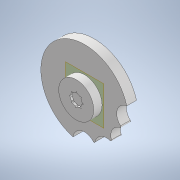
# Autodesk Inventor part: handle_base3
Saved by Autodesk Inventor 2021 (Build 250183000, 183)
## iProperties
Created: 2021-07-05
Part Number: handle_base3
Material: Generic
Document SubType Name: Modeling
Designer: teh18
Density: 1 g/cm^3
Appearance: Default
Author: teh18
Autodesk Inventor part; units mm, degrees
ref_plane "YZ Plane" through (0, 0, 0) normal (1, 0, 0) x (0, 1, 0)
ref_plane "XZ Plane" through (0, 0, 0) normal (0, 1, 0) x (-1, 0, 0)
ref_plane "XY Plane" through (0, 0, 0) normal (0, 0, 1) x (1, 0, 0)
sketch "Sketch1" plane through (0, 0, 0) normal (0, 0, 1) x (1, 0, 0)
  circle A0 centre (0, 0) radius 6
  circle A1 centre (0, 0) radius 20 projected
  circle A2 centre (0, 0) radius 5 projected
  arc A3 (6.0947, -0.2544) -> (5.2397, 3.1233) centre (0, 0) ccw projected
  arc A4 (4.1297, -4.4895) -> (5.9136, -1.4965) centre (0, 0) ccw projected
  arc A5 (-0.2544, -6.0947) -> (3.1233, -5.2397) centre (0, 0) ccw projected
  arc A6 (-4.4895, -4.1297) -> (-1.4965, -5.9136) centre (0, 0) ccw projected
  arc A7 (-6.0947, 0.2544) -> (-5.2397, -3.1233) centre (0, 0) ccw projected
  arc A8 (-4.1297, 4.4895) -> (-5.9136, 1.4965) centre (0, 0) ccw projected
  arc A9 (0.2544, 6.0947) -> (-3.1233, 5.2397) centre (0, 0) ccw projected
  arc A10 (4.4895, 4.1297) -> (1.4965, 5.9136) centre (0, 0) ccw projected
  line L0 (5.7362, 4.2762) -> (5.2397, 3.1233) projected
  line L1 (6.0947, -0.2544) -> (7.0798, -1.0323) projected
  line L2 (7.0798, -1.0323) -> (5.9136, -1.4965) projected
  line L3 (4.1297, -4.4895) -> (4.2762, -5.7362) projected
  line L4 (4.2762, -5.7362) -> (3.1233, -5.2397) projected
  line L5 (-0.2544, -6.0947) -> (-1.0323, -7.0798) projected
  line L6 (-1.0323, -7.0798) -> (-1.4965, -5.9136) projected
  line L7 (-4.4895, -4.1297) -> (-5.7362, -4.2762) projected
  line L8 (-5.7362, -4.2762) -> (-5.2397, -3.1233) projected
  line L9 (-6.0947, 0.2544) -> (-7.0798, 1.0323) projected
  line L10 (-7.0798, 1.0323) -> (-5.9136, 1.4965) projected
  line L11 (-4.1297, 4.4895) -> (-4.2762, 5.7362) projected
  line L12 (-4.2762, 5.7362) -> (-3.1233, 5.2397) projected
  line L13 (0.2544, 6.0947) -> (1.0323, 7.0798) projected
  line L14 (1.0323, 7.0798) -> (1.4965, 5.9136) projected
  line L15 (4.4895, 4.1297) -> (5.7362, 4.2762) projected
  line L16 (4.1567, -5.5758) -> (4.0244, -4.4502)
  arc A11 (4.0244, -4.4502) -> (5.8289, -1.4226) centre (0, 0) ccw
  line L17 (5.8289, -1.4226) -> (6.8819, -1.0035)
  line L18 (6.8819, -1.0035) -> (5.9924, -0.3011)
  arc A12 (5.9924, -0.3011) -> (5.1276, 3.1157) centre (0, 0) ccw
  line L19 (5.1276, 3.1157) -> (5.5758, 4.1567)
  line L20 (5.5758, 4.1567) -> (4.4502, 4.0244)
  arc A13 (4.4502, 4.0244) -> (1.4226, 5.8289) centre (0, 0) ccw
  line L21 (1.4226, 5.8289) -> (1.0035, 6.8819)
  line L22 (1.0035, 6.8819) -> (0.3011, 5.9924)
  arc A14 (0.3011, 5.9924) -> (-3.1157, 5.1276) centre (0, 0) ccw
  line L23 (-3.1157, 5.1276) -> (-4.1567, 5.5758)
  line L24 (-4.1567, 5.5758) -> (-4.0244, 4.4502)
  arc A15 (-4.0244, 4.4502) -> (-5.8289, 1.4226) centre (0, 0) ccw
  line L25 (-5.8289, 1.4226) -> (-6.8819, 1.0035)
  line L26 (-6.8819, 1.0035) -> (-5.9924, 0.3011)
  arc A16 (-5.9924, 0.3011) -> (-5.1276, -3.1157) centre (0, 0) ccw
  line L27 (-5.1276, -3.1157) -> (-5.5758, -4.1567)
  line L28 (-5.5758, -4.1567) -> (-4.4502, -4.0244)
  arc A17 (-4.4502, -4.0244) -> (-1.4226, -5.8289) centre (0, 0) ccw
  line L29 (-1.4226, -5.8289) -> (-1.0035, -6.8819)
  line L30 (-1.0035, -6.8819) -> (-0.3011, -5.9924)
  arc A18 (-0.3011, -5.9924) -> (3.1157, -5.1276) centre (0, 0) ccw
  line L31 (3.1157, -5.1276) -> (4.1567, -5.5758)
  point P0 (0, 0)
  point P1 (0, 0)
  point P2 (5.8289, -1.4226)
  point P3 (3.1157, -5.1276)
  point P4 (-1.4226, -5.8289)
  point P5 (-5.1276, -3.1157)
  point P6 (-5.8289, 1.4226)
  point P7 (-3.1157, 5.1276)
  point P8 (1.4226, 5.8289)
  point P9 (5.1276, 3.1157)
  dimension "d0" = 0.1
  dimension "d14" = 0.1
  constraints: 32 end point, 16 point on circle, 9 centre point, 23 other
  measures "d0" radial gap between concentric circles of A3 A0
  measures "d14" distance between parallel lines of L3 L16
extrude "Extrusion1" add sketch "Sketch1" against normal blind 10 contours A0 | A0 L20 L19 | L18 L17 A0 | A0 L22 L21 | L16 L31 A0 | A0 L24 L23 | L30 L29 A0 | A0 L26 L25 | L28 L27 A0
sketch "Sketch2" plane through (0, 0, 0) normal (0, 0, 1) x (-0.7848184, 0.6197258, 0)
  arc A0 (-4.8896, -3.4774) -> (-2.0933, -5.623) centre (0, 0) ccw projected
  circle A1 centre (0, 0) radius 18
  point P0 (0, 0)
  constraints: 1 centre point
extrude "Extrusion2" add sketch "Sketch2" along normal blind 20
sketch "Sketch6" plane through (0, 0, 20) normal (0, 0, 1) x (-0.6197258, -0.7848184, 0)
  arc A0 (4.2796, 4.2066) -> (1.664, 5.7655) centre (0, 0) ccw
  line L0 (4.2796, 4.2066) -> (5.8979, 4.3968)
  line L1 (5.8979, 4.3968) -> (5.2535, 2.9002)
  arc A1 (6.0006, -0.0517) -> (5.2535, 2.9002) centre (0, 0) ccw
  line L2 (6.0006, -0.0517) -> (7.2794, -1.0614)
  line L3 (7.2794, -1.0614) -> (5.7655, -1.664)
  arc A2 (4.2066, -4.2796) -> (5.7655, -1.664) centre (0, 0) ccw
  line L4 (4.2066, -4.2796) -> (4.3968, -5.8979)
  line L5 (4.3968, -5.8979) -> (2.9002, -5.2535)
  arc A3 (-0.0517, -6.0006) -> (2.9002, -5.2535) centre (0, 0) ccw
  line L6 (-0.0517, -6.0006) -> (-1.0614, -7.2794)
  line L7 (-1.0614, -7.2794) -> (-1.664, -5.7655)
  arc A4 (-4.2796, -4.2066) -> (-1.664, -5.7655) centre (0, 0) ccw
  line L8 (-4.2796, -4.2066) -> (-5.8979, -4.3968)
  line L9 (-5.8979, -4.3968) -> (-5.2535, -2.9002)
  arc A5 (-6.0006, 0.0517) -> (-5.2535, -2.9002) centre (0, 0) ccw
  line L10 (-6.0006, 0.0517) -> (-7.2794, 1.0614)
  line L11 (-7.2794, 1.0614) -> (-5.7655, 1.664)
  arc A6 (-4.2066, 4.2796) -> (-5.7655, 1.664) centre (0, 0) ccw
  line L12 (-4.2066, 4.2796) -> (-4.3968, 5.8979)
  line L13 (-4.3968, 5.8979) -> (-2.9002, 5.2535)
  arc A7 (0.0517, 6.0006) -> (-2.9002, 5.2535) centre (0, 0) ccw
  line L14 (0.0517, 6.0006) -> (1.0614, 7.2794)
  line L15 (1.0614, 7.2794) -> (1.664, 5.7655)
  point P0 (0, 0)
  constraints: 32 end point, 16 point on circle, 8 centre point
extrude "Extrusion5" cut sketch "Sketch6" against normal blind 2.1
ref_plane "Work Plane2" through (0, 0, 11.375) normal (0, 0, -1) x (-1, 0, 0)
sketch "Sketch9" plane through (0, 0, 11.375) normal (0, 0, -1) x (-1, 0, 0)
  circle A0 centre (-49.4955, -7.0845) radius 2.25 projected
  line L0 (-31.1338, -24.8496) -> (-45.3829, -4.241) projected
  arc A1 (-45.3829, -4.241) -> (-54.2408, -5.5088) centre (-49.4955, -7.0845) ccw projected
  line L1 (-54.2408, -5.5088) -> (-62.1365, -29.2871) projected
  arc A2 (-62.1365, -29.2871) -> (-52.3258, -50.9279) centre (-45.5282, -34.802) ccw projected
  line L2 (-52.3258, -50.9279) -> (-34.4799, -48.3735) projected
  arc A3 (-34.4799, -48.3735) -> (-31.1338, -24.8496) centre (-45.5282, -34.802) ccw projected
  circle A4 centre (-45.5282, -34.802) radius 12.5 projected
  circle A5 centre (0, 0) radius 18 projected
  circle A6 centre (-49.4955, -7.0845) radius 2.25 projected
  circle A7 centre (-49.4955, -7.0845) radius 12
  circle A8 centre (0, 0) radius 42.5
  arc A9 (-40.8059, -11.8798) -> (-40.8059, 11.8798) centre (-42.5, 0) ccw
  arc A10 (-29.399, -30.6912) -> (-41.2788, -10.1147) centre (-36.8061, -21.25) ccw
  arc A11 (-10.1147, -41.2788) -> (-30.6912, -29.399) centre (-21.25, -36.8061) ccw
  arc A12 (11.8798, -40.8059) -> (-11.8798, -40.8059) centre (0, -42.5) ccw
  point P0 (0, 0)
  point P1 (-9.3836, -35.0202)
  point P2 (11.8798, -40.8059)
  point P3 (-35.0202, -9.3836)
  point P4 (-25.6366, -25.6366)
  dimension "d16" = 24
  dimension "d17" = 85
  dimension "d21" = 90
  dimension "d26" = 12
  constraints: 11 point on circle, 6 centre point, 2 coincident, 13 other
  measures "d16" diameter of A7
  measures "d17" diameter of A8
  measures "d26" radius of A9
extrude "Extrusion6" add sketch "Sketch9" along normal blind 10 contours A10 A9 A8 A12 A11
fillet "Fillet1" radius 1 3 edges at (35.0202, -9.3836, 6.375) (25.6366, -25.6366, 6.375) (9.3836, -35.0202, 6.375)
body "Solid1"
